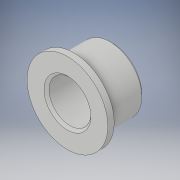
# Autodesk Inventor part: robotics
Saved by Autodesk Inventor 2017 (Build 210142000, 142)
## iProperties
Created: 2017-02-10
Part Number: robotics
Material: Generic
Document SubType Name: Modeling
Designer: margr
Density: 1 g/cm^3
Appearance: Default
Author: margr
Autodesk Inventor part; units mm, degrees
ref_plane "YZ Plane" through (0, 0, 0) normal (1, 0, 0) x (0, 1, 0)
ref_plane "XZ Plane" through (0, 0, 0) normal (0, 1, 0) x (-1, 0, 0)
ref_plane "XY Plane" through (0, 0, 0) normal (0, 0, 1) x (1, 0, 0)
sketch "Sketch1" plane through (0, 0, 0) normal (0, 0, 1) x (1, 0, 0)
  point P0 (0, 0)
sketch "Sketch2" plane through (0, 0, 0) normal (0, 0, 1) x (1, 0, 0)
  circle A0 centre (0, 0) radius 6.35
  circle A1 centre (0, 0) radius 4.1783
  dimension "d0" = 8.3566
  dimension "d1" = 12.7
  constraints: 2 centre point, 2 coincident
  measures "d0" diameter of A1
  measures "d1" diameter of A0
extrude "Extrusion1" add sketch "Sketch2" along normal blind 7.747
sketch "Sketch3" plane through (0, 0, 7.747) normal (0, 0, 1) x (1, 0, 0)
  circle A0 centre (0, 0) radius 4.1783 projected
  circle A1 centre (0, 0) radius 8.0645
  dimension "d4" = 16.129
  constraints: 1 centre point, 1 coincident
  measures "d4" diameter of A1
extrude "Extrusion2" add sketch "Sketch3" along normal blind 1.27
chamfer "Chamfer1" distance 0.508 angle 45 3 edges at (-4.1783, 0, 0) (-6.35, 0, 0) (-4.1783, 0, 9.017)
body "Solid1"
